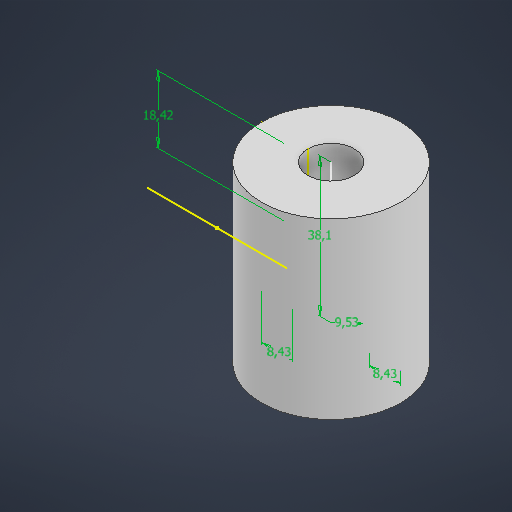
# Autodesk Inventor part: peca5
Saved by Autodesk Inventor 2026.2 (Build 302298000, 298)
## iProperties
Created: 2026-09-25
Part Number: peca5
Material: Genérico
Document SubType Name: Modeling
Designer: IFSP
Density: 1 g/cm^3
Appearance: Padrão
Author: IFSP
Autodesk Inventor part; units mm, degrees
ref_plane "YZ Plane" through (0, 0, 0) normal (1, 0, 0) x (0, 1, 0)
ref_plane "XZ Plane" through (0, 0, 0) normal (0, 1, 0) x (-1, 0, 0)
sketch "Esboço1" plane through (0, 0, 0) normal (0, 1, 0) x (-1, 0, 0)
  circle A0 centre (0, 0) radius 19.05
  circle A1 centre (0, 0) radius 6.35
  dimension "d0" = 38.1
  dimension "d1" = 12.7
  constraints: 2 centre point, 2 coincident
  measures "d0" diameter of A0
  measures "d1" diameter of A1
extrude "Extrusão1" add sketch "Esboço1" against normal blind 47.63
ref_plane "Plano de trabalho1" through (0, 0, 31.25) normal (0, 0, 1) x (1, 0, 0)
sketch "Esboço2" plane through (0, 0, 31.25) normal (0, 0, 1) x (1, 0, 0)
  line L0 (19.05, 0) -> (-19.05, 0) projected
  point P0 (0, 0)
sketch "Esboço3" plane through (0, 0, 0) normal (0, 0, 1) x (1, 0, 0)
  line L0 (-19.05, 0) -> (-19.05, -47.63) projected
  line L1 (-6.35, -47.63) -> (-6.35, 0) projected
  line L2 (19, -40) -> (10.57, -40)
  line L3 (-19, -40) -> (-10.57, -40)
  line L4 (-12.8553, -1.992) -> (-12.8553, -20.412)
  line L5 (0, 0) -> (0, -38.1)
  circle A0 centre (0, -38.1) radius 9.53
  dimension "d20" = 8.43
  dimension "d21" = 8.43
  dimension "d22" = 18.42
  dimension "d23" = 38.1
  dimension "d24" = 9.53
  constraints: 8 end point, 2 point on line, 2 vertical, 1 centre point, 1 coincident, 1 horizontal
  measures "d20" distance of L2.start L2.end
  measures "d21" distance of L3.start L3.end
  measures "d22" distance of L4.start L4.end
  measures "d23" distance of L5.start L5.end
  measures "d24" radius of A0
